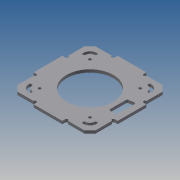
# Autodesk Inventor part: tapa ventilador
Saved by Autodesk Inventor 2017 (Build 210142000, 142)
## iProperties
Part Number: tapa ventilador
Material: Genérico
Document SubType Name: Modeling
Designer: Leo
Density: 1 g/cm^3
Appearance: Valor por defecto
Description: Aluminio compuesto routeado CNC
Author: Leo
Autodesk Inventor part; units mm, degrees
ref_plane "YZ Plane" through (0, 0, 0) normal (1, 0, 0) x (0, 1, 0)
ref_plane "XZ Plane" through (0, 0, 0) normal (0, 1, 0) x (-1, 0, 0)
ref_plane "XY Plane" through (0, 0, 0) normal (0, 0, 1) x (1, 0, 0)
sketch "Boceto1" plane through (0, 0, 0) normal (0, 0, 1) x (1, 0, 0)
  line L0 (35, 35) -> (-35, 35) construction
  line L1 (-35, 35) -> (-35, -35) construction
  line L2 (-35, -35) -> (35, -35) construction
  line L3 (35, -35) -> (35, 35) construction
  circle A0 centre (35, 35) radius 2
  circle A1 centre (35, -35) radius 2
  circle A2 centre (-35, -35) radius 2
  circle A3 centre (-35, 35) radius 2
  circle A4 centre (0, 0) radius 32.5
  line L4 (50, 12) -> (50, -12)
  arc A5 (47.6827, -13.9747) -> (50, -12) centre (48, -12) ccw
  line L5 (47.6827, -13.9747) -> (40.6827, -12.85)
  arc A6 (39, -10.8753) -> (40.6827, -12.85) centre (41, -10.8753) ccw
  line L6 (39, -10.8753) -> (39, 10.8753)
  arc A7 (40.6827, 12.85) -> (39, 10.8753) centre (41, 10.8753) ccw
  line L7 (40.6827, 12.85) -> (47.6827, 13.9747)
  arc A8 (50, 12) -> (47.6827, 13.9747) centre (48, 12) ccw
  line L8 (0, 7) -> (32, 7) construction
  line L9 (32, 7) -> (32, 31) construction
  line L10 (32, 31) -> (0, 31) construction
  line L11 (0, 31) -> (0, 7) construction
  line L12 (29.5, -31) -> (29.5, -12) construction
  line L13 (29.5, -12) -> (2.5, -12) construction
  line L14 (2.5, -12) -> (2.5, -31) construction
  line L15 (2.5, -31) -> (29.5, -31) construction
  arc A9 (-37.5, -47.6) -> (-37.5, -43.4) centre (-37.5, -45.5) ccw projected
  arc A10 (-43.4, -37.5) -> (-37.5, -43.4) centre (-37.5, -37.5) ccw projected
  arc A11 (-43.4, -37.5) -> (-47.6, -37.5) centre (-45.5, -37.5) ccw projected
  arc A12 (-47.6, -37.5) -> (-37.5, -47.6) centre (-37.5, -37.5) ccw projected
  arc A13 (-47.6, 37.5) -> (-43.4, 37.5) centre (-45.5, 37.5) ccw projected
  arc A14 (-37.5, 43.4) -> (-43.4, 37.5) centre (-37.5, 37.5) ccw projected
  arc A15 (-37.5, 43.4) -> (-37.5, 47.6) centre (-37.5, 45.5) ccw projected
  arc A16 (-37.5, 47.6) -> (-47.6, 37.5) centre (-37.5, 37.5) ccw projected
  arc A17 (37.5, 47.6) -> (37.5, 43.4) centre (37.5, 45.5) ccw projected
  arc A18 (43.4, 37.5) -> (37.5, 43.4) centre (37.5, 37.5) ccw projected
  arc A19 (43.4, 37.5) -> (47.6, 37.5) centre (45.5, 37.5) ccw projected
  arc A20 (47.6, 37.5) -> (37.5, 47.6) centre (37.5, 37.5) ccw projected
  arc A21 (37.5, -43.4) -> (37.5, -47.6) centre (37.5, -45.5) ccw projected
  arc A22 (37.5, -47.6) -> (47.6, -37.5) centre (37.5, -37.5) ccw projected
  arc A23 (47.6, -37.5) -> (43.4, -37.5) centre (45.5, -37.5) ccw projected
  arc A24 (37.5, -43.4) -> (43.4, -37.5) centre (37.5, -37.5) ccw projected
  line L16 (-58.5, 20) -> (-58.5, -20) projected
  line L17 (-54.5, 20) -> (-58.5, 20) projected
  arc A25 (-54.5, 20) -> (-54.5, 24) centre (-54.5, 22) ccw projected
  line L18 (-54.5, 46.5) -> (-54.5, 24) projected
  line L19 (-46.5, 54.5) -> (-54.5, 46.5) projected
  line L20 (-24, 54.5) -> (-46.5, 54.5) projected
  arc A26 (-24, 54.5) -> (-20, 54.5) centre (-22, 54.5) ccw projected
  line L21 (-20, 58.5) -> (-20, 54.5) projected
  line L22 (20, 58.5) -> (-20, 58.5) projected
  line L23 (20, 54.5) -> (20, 58.5) projected
  arc A27 (20, 54.5) -> (24, 54.5) centre (22, 54.5) ccw projected
  line L24 (46.5, 54.5) -> (24, 54.5) projected
  line L25 (54.5, 46.5) -> (46.5, 54.5) projected
  line L26 (54.5, 24) -> (54.5, 46.5) projected
  arc A28 (54.5, 24) -> (54.5, 20) centre (54.5, 22) ccw projected
  line L27 (58.5, 20) -> (54.5, 20) projected
  line L28 (58.5, -20) -> (58.5, 20) projected
  line L29 (54.5, -20) -> (58.5, -20) projected
  arc A29 (54.5, -20) -> (54.5, -24) centre (54.5, -22) ccw projected
  line L30 (54.5, -46.5) -> (54.5, -24) projected
  line L31 (46.5, -54.5) -> (54.5, -46.5) projected
  line L32 (24, -54.5) -> (46.5, -54.5) projected
  arc A30 (24, -54.5) -> (20, -54.5) centre (22, -54.5) ccw projected
  line L33 (20, -58.5) -> (20, -54.5) projected
  line L34 (-20, -58.5) -> (20, -58.5) projected
  line L35 (-20, -54.5) -> (-20, -58.5) projected
  arc A31 (-20, -54.5) -> (-24, -54.5) centre (-22, -54.5) ccw projected
  line L36 (-46.5, -54.5) -> (-24, -54.5) projected
  line L37 (-54.5, -46.5) -> (-46.5, -54.5) projected
  line L38 (-54.5, -24) -> (-54.5, -46.5) projected
  arc A32 (-54.5, -24) -> (-54.5, -20) centre (-54.5, -22) ccw projected
  line L39 (-58.5, -20) -> (-54.5, -20) projected
  point P0 (35, 0)
  point P1 (58.5, 0)
  point P2 (0, 35)
  point P3 (39, 0)
  point P4 (50, 0)
  dimension "d0" = 70
  dimension "d1" = 4
  dimension "d2" = 65
  dimension "d3" = 2
  dimension "d4" = 11
  dimension "d5" = 28
  dimension "d6" = 25.7
  dimension "d8" = 4
  constraints: 16 end point, 9 centre point, 8 point on circle, 8 tangent, 6 equal radius, 5 coincident, 4 horizontal alignment, 4 midpoint, 3 parallel, 2 perpendicular, 1 horizontal, 1 vertical, 1 vertical alignment
  measures "d0" distance of L0.start L0.end
  measures "d1" diameter of A0
  measures "d2" diameter of A4
  measures "d3" radius of A7
  measures "d4" distance between parallel lines of L4 L6
  measures "d6" distance of L7.start L5.end
  measures "d8" distance between parallel lines of L6 L3
extrude "Extrusión1" add sketch "Boceto1" along normal blind 4
